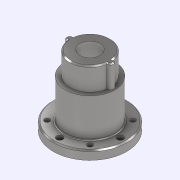
# Autodesk Inventor part: 18102021-002-09
Saved by Autodesk Inventor 2021 (Build 250183000, 183)
## iProperties
Created: 2021-10-17
Part Number: 18102021-002-09
Material: Stainless Steel
Document SubType Name: Modeling
Designer: DuctopwH
Density: 8 g/cm^3
Appearance: Semi-Polished
Author: DuctopwH
Autodesk Inventor part; units mm, degrees
ref_plane "YZ Plane" through (0, 0, 0) normal (1, 0, 0) x (0, 1, 0)
ref_plane "XZ Plane" through (0, 0, 0) normal (0, 1, 0) x (-1, 0, 0)
ref_plane "XY Plane" through (0, 0, 0) normal (0, 0, 1) x (1, 0, 0)
sketch "Sketch1" plane through (0, 0, 0) normal (0, 0, 1) x (1, 0, 0)
  line L0 (0, 0) -> (0, 22.9535)
  line L1 (12.5, 0) -> (12.5, 7)
  line L2 (12.5, 7) -> (8, 7)
  line L3 (8, 7) -> (8, 55.5)
  line L4 (8, 55.5) -> (16, 55.5)
  line L5 (16, 55.5) -> (16, 37.5)
  line L6 (16, 37.5) -> (19.5, 37.5)
  line L7 (19.5, 37.5) -> (19.5, 7)
  line L8 (19.5, 7) -> (29, 7)
  line L9 (29, 7) -> (29, 0)
  line L10 (29, 0) -> (12.5, 0)
  dimension "d0" = 25
  dimension "d1" = 16
  dimension "d2" = 32
  dimension "d3" = 55.5
  dimension "d4" = 30.5
  dimension "d5" = 7
  dimension "d6" = 58
  dimension "d7" = 7
  dimension "d8" = 39
  constraints: 22 end point, 9 perpendicular, 2 vertical, 1 point on line
  measures "d0" diameter of L1 L0
  measures "d1" diameter of L3 L0
  measures "d2" diameter of L5 L0
  measures "d3" distance between parallel lines of L10 L4
  measures "d4" distance between parallel lines of L8 L6
  measures "d5" distance between parallel lines of L10 L8
  measures "d6" diameter of L9 L0
  measures "d7" distance between parallel lines of L10 L2
  measures "d8" diameter of L7 L0
revolve "Revolution1" add sketch "Sketch1" angle 360 about axis through (0, 0, 0) along (0, 1, 0)
fillet "Fillet1" radius 1 1 edges at (-19.5, 7, 0)
sketch "Sketch2" plane through (0, 55.5, 0) normal (0, 1, 0) x (1, 0, 0)
  circle A0 centre (-16, 0) radius 2.5
  point P0 (0, 0)
  dimension "d11" = 5
  dimension "d12" = 16
  constraints: 1 centre point
  measures "d11" diameter of A0
  measures "d12" distance of point (0, 0) A0.centre
extrude "Extrusion1" add sketch "Sketch2" against normal up to surface (18 mm away)
mirror "Mirror1" about plane through (0, 0, 0) normal (1, 0, 0) of "Extrusion1"
chamfer "Chamfer1" distance 1 angle 45 5 edges at (0, 55.5, 16) (-18.5, 55.5, 0) (0, 55.5, -16) (18.5, 55.5, 0) (-29, 7, 0)
sketch "Sketch3" plane through (0, 7, 0) normal (0, 1, 0) x (1, 0, 0)
  circle A0 centre (0, 0) radius 24
  line L0 (-27.5, 0) -> (-20.5, 0)
  circle A1 centre (0, 0) radius 20.5 projected
  circle A2 centre (0, 0) radius 29 projected
  circle A3 centre (-24, 0) radius 2.5
  circle A4 centre (-16.9706, 16.9706) radius 2.065
  circle A5 centre (0, -24) radius 2.5
  circle A6 centre (-16.9706, -16.9706) radius 2.065
  circle A7 centre (24, 0) radius 2.5
  circle A8 centre (16.9706, -16.9706) radius 2.065
  circle A9 centre (0, 24) radius 2.5
  circle A10 centre (16.9706, 16.9706) radius 2.065
  line L1 (0, 0) -> (-16.9706, 16.9706)
  dimension "d19" = 5
  dimension "d20" = 4.13
  dimension "d23" = 360
  dimension "d27" = 24
  dimension "d28" = 45
  constraints: 9 centre point, 4 end point, 2 coincident, 2 point on circle, 1 horizontal, 1 horizontal alignment, 1 midpoint, 1 point on line, 18 other
  measures "d19" diameter of A3
  measures "d20" diameter of A4
  measures "d27" distance of point (0, 0) A3.centre
  measures "d28" angle of L0 L1
extrude "Extrusion2" cut sketch "Sketch3" against normal through all contours A0 A7 | A0 A7 | A10 A0 | A0 A10 | A8 A0 | A0 A8 | A9 A0 | A0 A9 | A5 A0 | A0 A5 | A4 L1 A0 | A0 A4 | A6 A0 | A0 A6 | L1 A4 A0 | A3 L0 A0 | A0 L0 A3 | A3 L0 A0 | A0 L0 A3
sketch "Sketch4" plane through (0, 55.5, 0) normal (0, 1, 0) x (1, 0, 0)
  line L0 (0, 48.5672) -> (-36.0767, 48.5672)
  line L1 (-36.0767, 48.5672) -> (-36.0767, -45.6507)
  line L2 (-36.0767, -45.6507) -> (0, -45.6507)
  line L3 (0, -45.6507) -> (0, 48.5672)
  point P0 (0, 0)
  constraints: 8 end point, 2 parallel, 1 horizontal, 1 perpendicular
body "Solid1"
